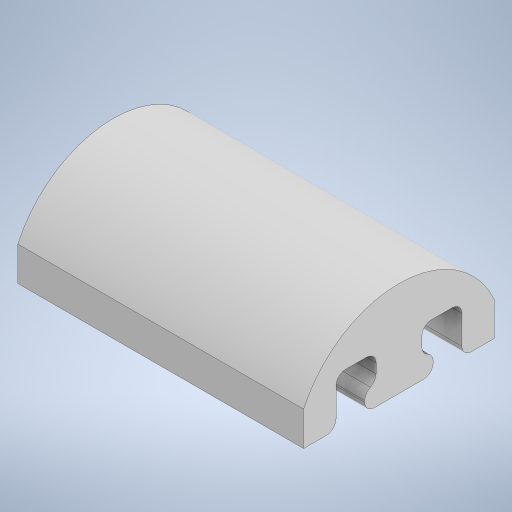
# Autodesk Inventor part: wciskacz_v2
Saved by Autodesk Inventor 2024.2 (Build 282272000, 272)
## iProperties
Created: 2024-01-13
Part Number: wciskacz_v2
Material: PLA
Document SubType Name: Modeling
Designer: Konrad
Density: 1 g/cm^3
Appearance: Domyślna
Author: Konrad
Autodesk Inventor part; units mm, degrees
ref_plane "YZ Plane" through (0, 0, 0) normal (1, 0, 0) x (0, 1, 0)
ref_plane "XZ Plane" through (0, 0, 0) normal (0, 1, 0) x (-1, 0, 0)
ref_plane "XY Plane" through (0, 0, 0) normal (0, 0, 1) x (1, 0, 0)
sketch "Szkic1" plane through (0, 0, 0) normal (1, 0, 0) x (0, 1, 0)
  line L0 (0, 0) -> (10, 0) construction
  line L1 (0, 0) -> (0, -3.6)
  line L2 (0, -3.6) -> (2, -3.6)
  line L3 (2, -3.6) -> (2, -2.4)
  line L4 (2, -2.4) -> (5, -2.4)
  line L5 (5, -2.4) -> (5, -6.6)
  line L6 (5, -6.6) -> (0, -6.6)
  arc A0 (3.5826, -10) -> (10, 0) centre (-1, 0) ccw
  line L7 (0, 0) -> (0, 3.6)
  line L8 (0, 3.6) -> (2, 3.6)
  line L9 (2, 3.6) -> (2, 2.4)
  line L10 (2, 2.4) -> (5, 2.4)
  line L11 (5, 2.4) -> (5, 6.6)
  line L12 (5, 6.6) -> (0, 6.6)
  arc A1 (10, 0) -> (3.5826, 10) centre (-1, 0) ccw
  line L13 (3.5826, -10) -> (0, -10)
  line L14 (0, -10) -> (0, -6.6)
  line L15 (0, 6.6) -> (0, 10)
  line L16 (0, 10) -> (3.5826, 10)
  dimension "d10" = 3.6
  dimension "d13" = 3
  dimension "d14" = 11
  dimension "d19" = 5
  dimension "d22" = 10
  dimension "d28" = 10
  dimension "d29" = 4.2
  dimension "d32" = 3
  dimension "d34" = 2
  constraints: 34 end point, 8 symmetric about line, 7 perpendicular, 4 point on circle, 2 centre point, 2 horizontal, 2 point on line, 1 coincident, 1 vertical, 1 other
  measures "d10" distance of L0.start L1.end
  measures "d13" distance of L3.end L4.end
  measures "d14" radius of A0
  measures "d19" distance of L12.start L12.end
  measures "d22" distance from line of L0 L15.end
  measures "d28" distance of L0.start L0.end
  measures "d29" distance of L4.end L5.end
  measures "d32" distance between parallel lines of L6 L2
  measures "d34" distance of L8.start L8.end
extrude "Wyciągnięcie proste1" add sketch "Szkic1" along normal blind 30
fillet "Zaokrąglenie2" radius 1 12 edges at (15, 5, -2.4) (15, 5, -6.6) (15, 2, -3.6) (15, 0, -3.6) (15, 0, 3.6) (15, 2, 3.6) (15, 2, 2.4) (15, 5, 2.4) (15, 5, 6.6) (15, 0, 6.6) (15, 0, -6.6) (15, 2, -2.4)
